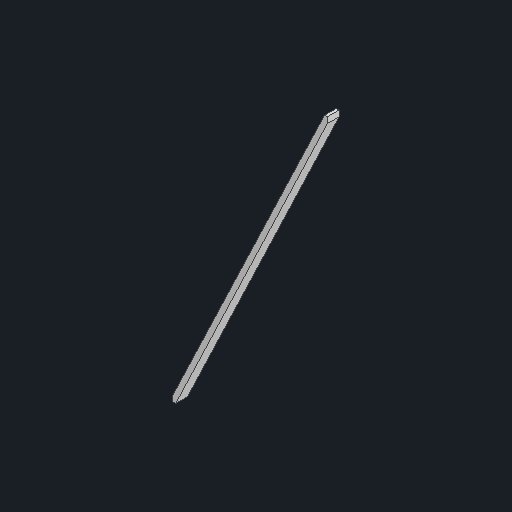
# Autodesk Inventor part: S_2x4x106.344
Saved by Autodesk Inventor 2026 (Build 300175000, 175)
## iProperties
Created: 2025-09-05
Part Number: S_2x4x106.344
Material: Generic
Document SubType Name: Modeling
Designer: trott
Density: 1 g/cm^3
Appearance: Default
Author: trott
Autodesk Inventor part; units mm, degrees
ref_plane "YZ Plane" through (0, 0, 0) normal (1, 0, 0) x (0, 1, 0)
ref_plane "XZ Plane" through (0, 0, 0) normal (0, 1, 0) x (-1, 0, 0)
ref_plane "XY Plane" through (0, 0, 0) normal (0, 0, 1) x (1, 0, 0)
sketch "Sketch1" plane through (0, 0, 0) normal (0, 0, 1) x (1, 0, 0)
  line L0 (-581.025, -1219.2) -> (581.025, -1219.2)
  line L1 (581.025, -1219.2) -> (581.025, 1219.2)
  line L2 (581.025, 1219.2) -> (-581.025, 1219.2)
  line L3 (-581.025, 1219.2) -> (-581.025, -1219.2)
  line L4 (-581.025, -1219.2) -> (581.025, 1219.2) construction
  line L5 (581.025, -1219.2) -> (-581.025, 1219.2) construction
  line L6 (581.025, 1219.2) -> (-581.025, -1219.2)
  line L7 (-563.828, -1227.3954) -> (-598.222, -1211.0046)
  line L8 (598.222, 1211.0046) -> (563.828, 1227.3954)
  line L9 (563.828, 1227.3954) -> (-598.222, -1211.0046)
  line L10 (-563.828, -1227.3954) -> (598.222, 1211.0046)
  point P0 (0, 0)
  point P1 (559.9223, 1219.2)
  point P2 (-581.025, -1174.919)
  point P3 (-559.9223, -1219.2)
  point P4 (581.025, 1174.919)
  dimension "d0" = 1162.05
  dimension "d1" = 2438.4
  dimension "d2" = 38.1
  dimension "d3" = 38.1
  constraints: 22 end point, 4 midpoint, 3 equal length, 3 perpendicular, 1 horizontal
  measures "d0" distance of L2.end L1.end
  measures "d1" distance of L0.end L1.end
  measures "d2" distance of L7.start L7.end
  measures "d3" distance of L8.start L8.end
extrude "Extrusion1" add sketch "Sketch1" along normal blind 88.9 contours L6 L1 L10 L0 | L3 L9 L2 L6
body "Solid1"
